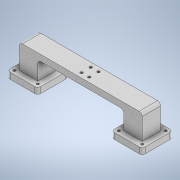
# Autodesk Inventor part: Platte für Gehäuse
Saved by Autodesk Inventor 2022 (Build 260153000, 153)
## iProperties
Created: 2023-01-30
Part Number: Platte für Gehäuse
Material: Stahl
Document SubType Name: Modeling
Designer: Matias Nicky
Density: 7.85 g/cm^3
Appearance: Aluminiumguss
Author: Matias Nicky
Autodesk Inventor part; units mm, degrees
ref_plane "YZ Plane" through (0, 0, 0) normal (1, 0, 0) x (0, 1, 0)
ref_plane "XZ Plane" through (0, 0, 0) normal (0, 1, 0) x (-1, 0, 0)
ref_plane "XY Plane" through (0, 0, 0) normal (0, 0, 1) x (1, 0, 0)
sketch "Skizze1" plane through (0, 0, 0) normal (0, 1, 0) x (-1, 0, 0)
  line L0 (-100, 15) -> (100, 15)
  line L1 (100, 15) -> (100, -15)
  line L2 (100, -15) -> (-100, -15)
  line L3 (-100, -15) -> (-100, 15)
  line L4 (-100, 15) -> (100, -15) construction
  line L5 (100, 15) -> (-100, -15) construction
  point P0 (0, 0)
  dimension "d0" = 30
  dimension "d1" = 200
  constraints: 12 end point, 2 midpoint, 2 parallel, 1 horizontal, 1 perpendicular
  measures "d0" distance between parallel lines of L2 L0
  measures "d1" distance between parallel lines of L3 L1
extrude "Extrusion1" add sketch "Skizze1" along normal blind 10
sketch "Skizze4" plane through (0, 10, 0) normal (0, 1, 0) x (1, 0, 0)
  line L0 (100, 15) -> (-100, 15) projected
  line L1 (100, -15) -> (100, 15) projected
  line L2 (-100, -15) -> (100, -15) projected
  line L3 (-100, 15) -> (-100, -15) projected
  line L4 (0, 21) -> (0, -21) projected
  point P0 (0, 0)
  point P1 (6.25, 7.5)
  point P2 (6.25, -7.5)
  point P3 (-6.25, -7.5)
  point P4 (-6.25, 7.5)
  dimension "d37" = 7.5
  dimension "d40" = 7.5
  dimension "d41" = 7.5
  dimension "d44" = 7.5
  dimension "d52" = 6.25
  dimension "d53" = 6.25
  dimension "d54" = 6.25
  dimension "d55" = 6.25
  measures "d37" distance from line of L0 point (6.25, 7.5)
  measures "d40" distance from line of L2 point (6.25, -7.5)
  measures "d41" distance from line of L0 point (-6.25, 7.5)
  measures "d44" distance from line of L2 point (-6.25, -7.5)
  measures "d52" distance from line of L4 point (6.25, 7.5)
  measures "d53" distance from line of L4 point (-6.25, 7.5)
  measures "d54" distance from line of L4 point (6.25, -7.5)
  measures "d55" distance from line of L4 point (-6.25, -7.5)
hole "Bohrung3" at (6.25, 10, -7.5) at (6.25, 10, 7.5) at (-6.25, 10, 7.5) at (-6.25, 10, -7.5) direction (0, -1, 0) diameter 4.134 depth 14.2 thread size "M5x0.8" class "6H" standard "ANSI Metric M Profile"
sketch "Skizze5" plane through (0, 0, 0) normal (0, -1, 0) x (1, 0, 0)
  line L0 (-100, 15) -> (100, 15) projected
  line L1 (-70, -15) -> (-100, -15)
  line L2 (-100, -15) -> (-100, 15)
  line L3 (-100, 15) -> (-70, 15)
  line L4 (-70, 15) -> (-70, -15)
  line L5 (-70, -15) -> (-100, 15) construction
  line L6 (-100, -15) -> (-70, 15) construction
  line L7 (-100, -15) -> (-100, 15) projected
  line L8 (100, -15) -> (-100, -15) projected
  line L9 (70, -15) -> (100, -15)
  line L10 (100, -15) -> (100, 15)
  line L11 (100, 15) -> (70, 15)
  line L12 (70, 15) -> (70, -15)
  line L13 (70, -15) -> (100, 15) construction
  line L14 (100, -15) -> (70, 15) construction
  line L15 (100, 15) -> (100, -15) projected
  point P0 (0, 0)
  point P1 (-12.5, 15)
  point P2 (-85, 0)
  point P3 (-12.5, -15)
  point P4 (85, 0)
  dimension "d56" = 0
  dimension "d57" = 0
  dimension "d58" = 30
  dimension "d59" = 30
  dimension "d60" = 30
  dimension "d61" = 0
  constraints: 24 end point, 4 midpoint, 4 parallel, 2 horizontal, 2 perpendicular, 1 point on line
  measures "d56" distance between parallel lines of L7 L2
  measures "d57" distance between parallel lines of L8 L1
  measures "d58" distance of L1.start L1.end
  measures "d59" distance of L11.end L10.end
  measures "d60" distance of L9.end L10.end
  measures "d61" distance between parallel lines of L15 L10
extrude "Extrusion3" add sketch "Skizze5" along normal blind 30 contours L0 L4 L1 L2 | L0 L10 L8 L12
sketch "Skizze6" plane through (0, -30, 0) normal (0, -1, 0) x (1, 0, 0)
  line L0 (-110, -25) -> (-60, -25)
  line L1 (-60, -25) -> (-60, 25)
  line L2 (-60, 25) -> (-110, 25)
  line L3 (-110, 25) -> (-110, -25)
  line L4 (-110, -25) -> (-60, 25) construction
  line L5 (-60, -25) -> (-110, 25) construction
  line L6 (-70, -15) -> (-70, 15) projected
  line L7 (60, 25) -> (110, 25)
  line L8 (110, 25) -> (110, -25)
  line L9 (110, -25) -> (60, -25)
  line L10 (60, -25) -> (60, 25)
  line L11 (60, 25) -> (110, -25) construction
  line L12 (110, 25) -> (60, -25) construction
  line L13 (100, -15) -> (100, 15) projected
  point P0 (0, 0)
  point P1 (-85, 0)
  point P2 (85, 0)
  dimension "d64" = 15
  dimension "d65" = 50
  dimension "d66" = 50
  dimension "d67" = 15
  dimension "d86" = 50
  dimension "d87" = 50
  constraints: 24 end point, 4 midpoint, 4 parallel, 2 horizontal, 2 perpendicular
  measures "d64" distance from line of L6 point (-85, 0)
  measures "d65" distance of L8.end L9.end
  measures "d66" distance of L7.end L8.end
  measures "d67" distance from line of L13 point (85, 0)
  measures "d86" distance of L1.end L2.end
  measures "d87" distance of L2.end L0.start
extrude "Extrusion4" add sketch "Skizze6" along normal blind 10
fillet "Rundung1" radius 5 8 edges at (-110, -35, 25) (-60, -35, 25) (-110, -35, -25) (-60, -35, -25) (60, -35, -25) (110, -35, -25) (110, -35, 25) (60, -35, 25)
sketch "Skizze7" plane through (0, -30, 0) normal (0, 1, 0) x (1, 0, 0)
  line L0 (110, 20) -> (110, -20) projected
  line L1 (105, -25) -> (65, -25) projected
  line L2 (60, -20) -> (60, 20) projected
  line L3 (65, 25) -> (105, 25) projected
  line L4 (-60, 20) -> (-60, -20) projected
  line L5 (-65, -25) -> (-105, -25) projected
  line L6 (-110, -20) -> (-110, 20) projected
  line L7 (-105, 25) -> (-65, 25) projected
  point P0 (0, 0)
  point P1 (104, -19)
  point P2 (66, -19)
  point P3 (66, 19)
  point P4 (104, 19)
  point P5 (-66, -19)
  point P6 (-104, -19)
  point P7 (-104, 19)
  point P8 (-66, 19)
  dimension "d71" = 6
  dimension "d72" = 6
  dimension "d73" = 6
  dimension "d74" = 6
  dimension "d75" = 6
  dimension "d76" = 6
  dimension "d77" = 6
  dimension "d78" = 6
  dimension "d79" = 6
  dimension "d80" = 6
  dimension "d81" = 6
  dimension "d82" = 6
  dimension "d83" = 6
  dimension "d84" = 6
  dimension "d85" = 6
  dimension "d95" = 6
  measures "d71" distance from line of L0 point (104, -19)
  measures "d72" distance from line of L1 point (104, -19)
  measures "d73" distance from line of L2 point (66, -19)
  measures "d74" distance from line of L1 point (66, -19)
  measures "d75" distance from line of L3 point (104, 19)
  measures "d76" distance from line of L0 point (104, 19)
  measures "d77" distance from line of L3 point (66, 19)
  measures "d78" distance from line of L2 point (66, 19)
  measures "d79" distance from line of point (-66, -19) L4
  measures "d80" distance from line of L5 point (-66, -19)
  measures "d81" distance from line of L5 point (-104, -19)
  measures "d82" distance from line of L6 point (-104, -19)
  measures "d83" distance from line of L6 point (-104, 19)
  measures "d84" distance from line of L7 point (-66, 19)
  measures "d85" distance from line of L4 point (-66, 19)
  measures "d95" distance from line of L7 point (-104, 19)
hole "Bohrung4" at (-66, -30, 19) at (104, -30, 19) at (104, -30, -19) at (66, -30, -19) at (66, -30, 19) at (-104, -30, 19) at (-66, -30, -19) at (-104, -30, -19) direction (0, -1, 0) diameter 4.134 depth 14.2 thread size "M5x0.8" class "6H" standard "ANSI Metric M Profile"
fillet "Rundung2" radius 5 4 edges at (100, 10, 0) (-100, 10, 0) (70, 0, 0) (-70, 0, 0)
equation "\"d46\" = d42"
equation "\"d89\" = d83"
equation "\"d42\" = 6.5"
